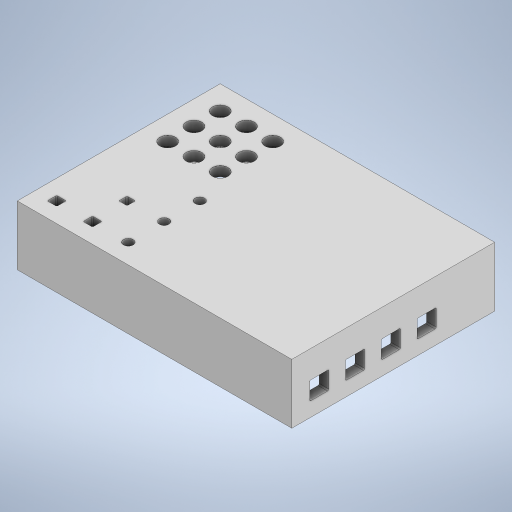
# Autodesk Inventor part: BreakoutBox
Saved by Autodesk Inventor 2023 (Build 270158000, 158)
## iProperties
Created: 2023-04-03
Part Number: BreakoutBox
Material: Generic
Document SubType Name: Modeling
Designer: yousefi
Density: 1 g/cm^3
Appearance: Default
Author: yousefi
Autodesk Inventor part; units mm, degrees
ref_plane "YZ Plane" through (0, 0, 0) normal (1, 0, 0) x (0, 1, 0)
ref_plane "XZ Plane" through (0, 0, 0) normal (0, 1, 0) x (-1, 0, 0)
ref_plane "XY Plane" through (0, 0, 0) normal (0, 0, 1) x (1, 0, 0)
sketch "main box1" plane through (0, 0, 0) normal (0, 1, 0) x (-1, 0, 0)
  line L0 (11.2873, -1.2021) -> (241.2873, -1.2021)
  line L1 (241.2873, -1.2021) -> (241.2873, -171.2021)
  line L2 (241.2873, -171.2021) -> (11.2873, -171.2021)
  line L3 (11.2873, -171.2021) -> (11.2873, -1.2021)
  point P0 (0, 0)
  dimension "d2" = 230
  dimension "d3" = 170
  constraints: 8 end point, 2 parallel, 1 horizontal, 1 perpendicular
  measures "d2" distance of L1.end L2.end
  measures "d3" distance of L0.end L1.end
extrude "Main box" add sketch "main box1" along normal blind 50
sketch "Ethernet1" plane through (-11.2873, 0, -1.2021) normal (1, 0, 0) x (0, 0, -1)
  line L0 (16, 27.2) -> (30, 27.2)
  line L1 (31, 26.2) -> (31, 13)
  line L2 (30, 12) -> (16, 12)
  line L3 (15, 13) -> (15, 26.2)
  line L4 (0, 0) -> (170, 0) projected
  line L5 (0, 0) -> (0, 50) projected
  arc A0 (16, 27.2) -> (15, 26.2) centre (16, 26.2) ccw
  arc A1 (15, 13) -> (16, 12) centre (16, 13) ccw
  arc A2 (30, 12) -> (31, 13) centre (30, 13) ccw
  arc A3 (31, 26.2) -> (30, 27.2) centre (30, 26.2) ccw
  line L6 (46, 27.2) -> (60, 27.2)
  line L7 (61, 26.2) -> (61, 13)
  line L8 (60, 12) -> (46, 12)
  line L9 (45, 13) -> (45, 26.2)
  arc A4 (46, 27.2) -> (45, 26.2) centre (46, 26.2) ccw
  arc A5 (45, 13) -> (46, 12) centre (46, 13) ccw
  arc A6 (60, 12) -> (61, 13) centre (60, 13) ccw
  arc A7 (61, 26.2) -> (60, 27.2) centre (60, 26.2) ccw
  arc A8 (76, 27.2) -> (75, 26.2) centre (76, 26.2) ccw
  arc A9 (75, 13) -> (76, 12) centre (76, 13) ccw
  line L10 (76, 27.2) -> (90, 27.2)
  arc A10 (91, 26.2) -> (90, 27.2) centre (90, 26.2) ccw
  line L11 (91, 26.2) -> (91, 13)
  line L12 (90, 12) -> (76, 12)
  arc A11 (90, 12) -> (91, 13) centre (90, 13) ccw
  line L13 (75, 13) -> (75, 26.2)
  arc A12 (106, 27.2) -> (105, 26.2) centre (106, 26.2) ccw
  line L14 (105, 13) -> (105, 26.2)
  arc A13 (105, 13) -> (106, 12) centre (106, 13) ccw
  line L15 (106, 27.2) -> (120, 27.2)
  line L16 (120, 12) -> (106, 12)
  arc A14 (121, 26.2) -> (120, 27.2) centre (120, 26.2) ccw
  line L17 (121, 26.2) -> (121, 13)
  arc A15 (120, 12) -> (121, 13) centre (120, 13) ccw
  point P0 (-1.2021, 0)
  point P1 (15, 27.2)
  point P2 (31, 12)
  point P3 (31, 27.2)
  point P4 (15, 12)
  point P5 (45, 27.2)
  point P6 (61, 12)
  point P7 (61, 27.2)
  point P8 (45, 12)
  point P9 (0, 25)
  point P10 (75, 27.2)
  point P11 (91, 27.2)
  point P12 (91, 12)
  point P13 (75, 12)
  point P14 (105, 27.2)
  point P15 (105, 12)
  point P16 (121, 27.2)
  point P17 (121, 12)
  dimension "d6" = 16
  dimension "d7" = 15.2
  dimension "d98" = 12
  dimension "d99" = 15
  dimension "d100" = 1
  dimension "d103" = 1
  dimension "d104" = 45
  dimension "d107" = 1
  dimension "d110" = 1
  dimension "d111" = 75
  dimension "d112" = 105
  constraints: 32 end point, 32 point on circle, 32 point on line, 32 tangent, 16 centre point, 12 equal radius, 9 collinear, 8 parallel, 4 horizontal, 4 perpendicular, 1 midpoint
  measures "d6" distance of point (31, 12) point (15, 12)
  measures "d7" distance of point (31, 27.2) point (31, 12)
  measures "d98" distance between parallel lines of L2 L4
  measures "d99" distance between parallel lines of L5 L3
  measures "d100" radius of A0
  measures "d103" radius of A4
  measures "d104" distance from line of point (0, 25) L9
  measures "d107" radius of A8
  measures "d110" radius of A12
  measures "d111" distance between parallel lines of L5 L13
  measures "d112" distance between parallel lines of L14 L5
extrude "Ethernet" cut sketch "Ethernet1" against normal blind 20
sketch "wheel 4 port connection" plane through (0, 50, 0) normal (0, 1, 0) x (1, 0, 0)
  line L0 (-221.7873, 21.7021) -> (-227.7873, 21.7021)
  line L1 (-228.7873, 20.7021) -> (-228.7873, 14.7021)
  line L2 (-227.7873, 13.7021) -> (-221.7873, 13.7021)
  line L3 (-220.7873, 14.7021) -> (-220.7873, 20.7021)
  line L4 (-241.2873, 171.2021) -> (-241.2873, 1.2021) projected
  line L5 (-241.2873, 1.2021) -> (-11.2873, 1.2021) projected
  arc A0 (-227.7873, 21.7021) -> (-228.7873, 20.7021) centre (-227.7873, 20.7021) ccw
  arc A1 (-220.7873, 20.7021) -> (-221.7873, 21.7021) centre (-221.7873, 20.7021) ccw
  arc A2 (-221.7873, 13.7021) -> (-220.7873, 14.7021) centre (-221.7873, 14.7021) ccw
  arc A3 (-228.7873, 14.7021) -> (-227.7873, 13.7021) centre (-227.7873, 14.7021) ccw
  point P0 (0, 0)
  point P1 (-220.7873, 21.7021)
  point P2 (-228.7873, 13.7021)
  point P3 (-228.7873, 21.7021)
  point P4 (-220.7873, 13.7021)
  dimension "d22" = 8
  dimension "d23" = 8
  dimension "d76" = 12.5
  dimension "d77" = 12.5
  dimension "d113" = 1
  constraints: 8 end point, 8 point on circle, 8 point on line, 8 tangent, 4 centre point, 3 equal radius, 2 parallel, 1 horizontal, 1 perpendicular
  measures "d22" distance of point (-220.787, 13.702) point (-228.787, 13.702)
  measures "d23" distance of point (-228.787, 13.702) point (-228.787, 21.702)
  measures "d76" distance between parallel lines of L1 L4
  measures "d77" distance between parallel lines of L5 L2
  measures "d113" radius of A0
extrude "wheel" cut sketch "wheel 4 port connection" against normal blind 20
sketch "Motor left 4 port connection" plane through (0, 50, 0) normal (0, 1, 0) x (1, 0, 0)
  line L0 (-191.7873, 21.7021) -> (-197.7873, 21.7021)
  line L1 (-198.7873, 20.7021) -> (-198.7873, 14.7021)
  line L2 (-197.7873, 13.7021) -> (-191.7873, 13.7021)
  line L3 (-190.7873, 14.7021) -> (-190.7873, 20.7021)
  line L4 (-241.2873, 1.2021) -> (-11.2873, 1.2021) projected
  line L5 (-220.7873, 20.7021) -> (-220.7873, 14.7021) projected
  arc A0 (-190.7873, 20.7021) -> (-191.7873, 21.7021) centre (-191.7873, 20.7021) ccw
  arc A1 (-191.7873, 13.7021) -> (-190.7873, 14.7021) centre (-191.7873, 14.7021) ccw
  arc A2 (-198.7873, 14.7021) -> (-197.7873, 13.7021) centre (-197.7873, 14.7021) ccw
  arc A3 (-197.7873, 21.7021) -> (-198.7873, 20.7021) centre (-197.7873, 20.7021) ccw
  point P0 (0, 0)
  point P1 (-190.7873, 21.7021)
  point P2 (-198.7873, 13.7021)
  point P3 (-198.7873, 21.7021)
  point P4 (-190.7873, 13.7021)
  point P5 (-221.7873, 20.7021)
  point P6 (-221.7873, 13.7021)
  dimension "d26" = 8
  dimension "d27" = 8
  dimension "d78" = 12.5
  dimension "d79" = 22
  dimension "d114" = 1
  constraints: 8 end point, 8 point on circle, 8 point on line, 8 tangent, 4 centre point, 3 equal radius, 2 parallel, 1 horizontal, 1 perpendicular, 1 other
  measures "d26" distance of point (-190.787, 13.702) point (-198.787, 13.702)
  measures "d27" distance of point (-198.787, 13.702) point (-198.787, 21.702)
  measures "d78" distance between parallel lines of L4 L2
  measures "d114" radius of A0
extrude "Motor left" cut sketch "Motor left 4 port connection" against normal blind 20
sketch "Motor right 4 port connection" plane through (0, 50, 0) normal (0, 1, 0) x (1, 0, 0)
  line L0 (-197.7873, 43.7021) -> (-192.7873, 43.7021)
  line L1 (-191.7873, 44.7021) -> (-191.7873, 49.7021)
  line L2 (-192.7873, 50.7021) -> (-197.7873, 50.7021)
  line L3 (-198.7873, 49.7021) -> (-198.7873, 44.7021)
  line L4 (-197.7873, 21.7021) -> (-191.7873, 21.7021) projected
  line L5 (-198.7873, 14.7021) -> (-198.7873, 20.7021) projected
  arc A0 (-197.7873, 50.7021) -> (-198.7873, 49.7021) centre (-197.7873, 49.7021) ccw
  arc A1 (-191.7873, 49.7021) -> (-192.7873, 50.7021) centre (-192.7873, 49.7021) ccw
  arc A2 (-192.7873, 43.7021) -> (-191.7873, 44.7021) centre (-192.7873, 44.7021) ccw
  arc A3 (-198.7873, 44.7021) -> (-197.7873, 43.7021) centre (-197.7873, 44.7021) ccw
  point P0 (0, 0)
  point P1 (-198.7873, 43.7021)
  point P2 (-191.7873, 50.7021)
  point P3 (-191.7873, 43.7021)
  point P4 (-198.7873, 50.7021)
  point P5 (-198.7873, 20.7021)
  point P6 (-191.7873, 20.7021)
  point P7 (-198.7873, 13.7021)
  dimension "d30" = 7
  dimension "d31" = 7
  dimension "d80" = 22
  dimension "d115" = 1
  constraints: 8 end point, 8 point on circle, 8 point on line, 8 tangent, 4 centre point, 3 equal radius, 2 parallel, 1 collinear, 1 horizontal, 1 perpendicular, 1 other
  measures "d30" distance of point (-198.787, 50.702) point (-191.787, 50.702)
  measures "d31" distance of point (-191.787, 50.702) point (-191.787, 43.702)
  measures "d115" radius of A0
extrude "Motor right" cut sketch "Motor right 4 port connection" against normal blind 20
sketch "Sketch10" plane through (0, 50, 0) normal (0, 1, 0) x (1, 0, 0)
  circle A0 centre (-164.7873, 17.7021) radius 4
  line L0 (-241.2873, 1.2021) -> (-11.2873, 1.2021) projected
  circle A1 centre (-164.7873, 47.7021) radius 4
  circle A2 centre (-164.7873, 77.7021) radius 4
  line L1 (-164.7873, 17.7021) -> (-164.7873, 77.7021) construction
  line L2 (-191.7873, 13.7021) -> (-197.7873, 13.7021) construction
  line L3 (-190.7873, 20.7021) -> (-190.7873, 14.7021) construction
  line L4 (-190.7873, 17.7021) -> (-164.7873, 17.7021) construction
  arc A3 (-198.7873, 14.7021) -> (-197.7873, 13.7021) centre (-197.7873, 14.7021) ccw construction
  arc A4 (-197.7873, 21.7021) -> (-198.7873, 20.7021) centre (-197.7873, 20.7021) ccw construction
  line L5 (-198.7873, 14.7021) -> (-198.7873, 20.7021) construction
  arc A5 (-198.7873, 14.7021) -> (-197.7873, 13.7021) centre (-197.7873, 14.7021) ccw construction
  line L6 (-191.7873, 13.7021) -> (-197.7873, 13.7021) construction
  arc A6 (-191.7873, 13.7021) -> (-190.7873, 14.7021) centre (-191.7873, 14.7021) ccw construction
  line L7 (-190.7873, 20.7021) -> (-190.7873, 14.7021) construction
  arc A7 (-190.7873, 20.7021) -> (-191.7873, 21.7021) centre (-191.7873, 20.7021) ccw construction
  line L8 (-197.7873, 21.7021) -> (-191.7873, 21.7021) construction
  point P0 (0, 0)
  point P1 (-194.7873, 13.7021)
  point P2 (-194.7873, 13.7021)
  dimension "d34" = 8
  dimension "d86" = 30
  dimension "d87" = 30
  dimension "d88" = 30
  constraints: 4 end point, 4 midpoint, 3 centre point, 2 equal radius, 1 perpendicular, 1 vertical
  measures "d34" diameter of A0
  measures "d86" distance of L1.start A1.centre
  measures "d87" distance of L1.end A1.centre
  measures "d88" horizontal distance of L1.start point (-194.787, 13.702)
extrude "PD" cut sketch "Sketch10" against normal blind 20
sketch "Power socket" plane through (0, 50, 0) normal (0, 1, 0) x (1, 0, 0)
  circle A0 centre (-221.2873, 107.2021) radius 6.5
  line L0 (-241.2873, 171.2021) -> (-241.2873, 1.2021) projected
  circle A1 centre (-221.2873, 129.2021) radius 6.5
  circle A2 centre (-221.2873, 151.2021) radius 6.5
  circle A3 centre (-199.2873, 151.2021) radius 6.5
  circle A4 centre (-199.2873, 129.2021) radius 6.5
  circle A5 centre (-199.2873, 107.2021) radius 6.5
  circle A6 centre (-177.2873, 151.2021) radius 6.5
  circle A7 centre (-177.2873, 129.2021) radius 6.5
  circle A8 centre (-177.2873, 107.2021) radius 6.5
  line L1 (-11.2873, 171.2021) -> (-241.2873, 171.2021) projected
  line L2 (-221.2873, 107.2021) -> (-221.2873, 151.2021) construction
  line L3 (-221.2873, 151.2021) -> (-177.2873, 151.2021) construction
  line L4 (-177.2873, 151.2021) -> (-177.2873, 107.2021) construction
  line L5 (-177.2873, 107.2021) -> (-221.2873, 107.2021) construction
  line L6 (-221.2873, 129.2021) -> (-177.2873, 129.2021) construction
  line L7 (-199.2873, 151.2021) -> (-199.2873, 107.2021) construction
  point P0 (0, 0)
  dimension "d43" = 13
  dimension "d90" = 20
  dimension "d94" = 20
  dimension "d95" = 22
  dimension "d96" = 22
  constraints: 12 end point, 9 centre point, 8 equal radius, 6 midpoint, 5 perpendicular, 3 coincident, 1 vertical
  measures "d43" diameter of A0
  measures "d90" distance from line of L0 L2.start
  measures "d94" distance from line of L1 A2.centre
  measures "d95" distance of L6.start A2.centre
  measures "d96" distance of L7.start A2.centre
extrude "Power" cut sketch "Power socket" against normal blind 20
sketch "Sketch22" plane through (0, 0, 0) normal (0, -1, 0) x (1, 0, 0)
  line L0 (-19.2873, -9.2021) -> (-233.2873, -9.2021)
  line L1 (-233.2873, -9.2021) -> (-233.2873, -163.2021)
  line L2 (-233.2873, -163.2021) -> (-19.2873, -163.2021)
  line L3 (-19.2873, -163.2021) -> (-19.2873, -9.2021)
  line L4 (-241.2873, -1.2021) -> (-11.2873, -1.2021) projected
  line L5 (-11.2873, -171.2021) -> (-241.2873, -171.2021) projected
  line L6 (-11.2873, -1.2021) -> (-11.2873, -171.2021) projected
  line L7 (-241.2873, -171.2021) -> (-241.2873, -1.2021) projected
  point P0 (0, 0)
  dimension "d70" = 8
  dimension "d71" = 8
  dimension "d72" = 8
  dimension "d73" = 8
  constraints: 8 end point, 2 parallel, 1 horizontal, 1 perpendicular
  measures "d70" distance between parallel lines of L4 L0
  measures "d71" distance between parallel lines of L5 L2
  measures "d72" distance between parallel lines of L6 L3
  measures "d73" distance between parallel lines of L7 L1
extrude "Extrusion21" cut sketch "Sketch22" against normal blind 42 contours L3 L2 L1 L0
body "Solid1"
